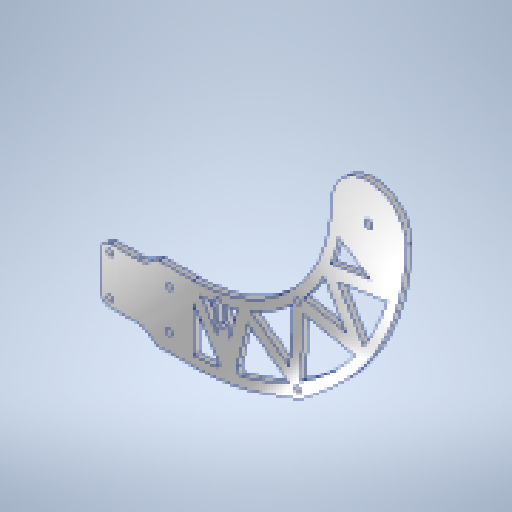
# Autodesk Inventor part: link1plate5
Saved by Autodesk Inventor 2024 (Build 280153000, 153)
## iProperties
Created: 2025-02-12
Part Number: link1plate5
Material: アルミニウム 6061
Document SubType Name: Modeling
Designer: tanoue_kota
Density: 2.7 g/cm^3
Appearance: アルミニウム - フラット
Mass: 39.1367 g
Surface Area: 135.061 cm^2
Volume: 14.4951 cm^3
Author: tanoue_kota
Autodesk Inventor part; units mm, degrees
ref_plane "YZ Plane" through (0, 0, 0) normal (1, 0, 0) x (0, 1, 0)
ref_plane "XZ Plane" through (0, 0, 0) normal (0, 1, 0) x (-1, 0, 0)
ref_plane "XY Plane" through (0, 0, 0) normal (0, 0, 1) x (1, 0, 0)
sketch "スケッチ1" plane through (0, 0, 0) normal (0, 0, 1) x (1, 0, 0)
  line L0 (0, 0) -> (-413, 0)
  line L1 (-413, 0) -> (-413, 19)
  line L2 (-413, 19) -> (0, 19)
  line L3 (0, 19) -> (0, 0)
  line L4 (-12.5, 0) -> (-47.5, 0)
  line L5 (-47.5, 0) -> (-47.5, 19)
  line L6 (-47.5, 19) -> (-12.5, 19)
  line L7 (-12.5, 19) -> (-12.5, 0)
  circle A0 centre (-413, 0) radius 510
  line L8 (-413, 0) -> (89.252, 88.5606)
  line L9 (89.252, 88.5606) -> (-410.748, 88.5606)
  line L10 (0, 0) -> (-20, 0)
  line L11 (-20, 0) -> (-20, 53.1786)
  line L12 (-20, 53.1786) -> (0, 53.1786)
  line L13 (0, 53.1786) -> (0, 0)
  line L14 (0, 53.1786) -> (-20, 53.1786)
  line L15 (-20, 53.1786) -> (-20, 88.5606)
  line L16 (-20, 88.5606) -> (0, 88.5606)
  line L17 (0, 88.5606) -> (0, 53.1786)
  circle A1 centre (89.252, 88.5606) radius 19
  line L18 (-413, -19) -> (0, -19)
  line L19 (0, -19) -> (0, 0)
  line L20 (-47.5, 0) -> (-47.5, -19)
  line L21 (-20, 0) -> (-20, -53.1786)
  line L22 (0, -53.1786) -> (0, 0)
  line L23 (0, -53.1786) -> (-20, -53.1786)
  line L24 (-413, 0) -> (-413, -19)
  arc A2 (0, 19) -> (70.2525, 88.7083) centre (0, 89.2547) ccw
  arc A3 (0, -19) -> (108.2514, 88.4128) centre (0, 89.2547) ccw
  line L25 (-47.5, 14) -> (-20, 14)
  line L26 (-47.5, -14) -> (-20, -14)
  line L27 (0, 88.5606) -> (6, 88.5606)
  line L28 (6, 88.5606) -> (6, 61.5606)
  line L29 (6, 61.5606) -> (0, 61.5606)
  line L30 (0, 61.5606) -> (0, 88.5606)
  line L31 (6, 88.5606) -> (57, 88.5606)
  line L32 (57, 88.5606) -> (57, 63.0606)
  line L33 (57, 63.0606) -> (6, 63.0606)
  line L34 (6, 63.0606) -> (6, 88.5606)
  line L35 (89.252, 88.5606) -> (0, 89.2547)
  point P0 (-20, 19)
  point P1 (-20, -14)
  point P2 (-20, -19)
  dimension "d4" = 1020
  dimension "d0" = 413
  dimension "d1" = 19
  dimension "d2" = 12.5
  dimension "d3" = 35
  dimension "d5" = 10
  dimension "d6" = 500
  dimension "d7" = 20
  dimension "d9" = 38
  dimension "d11" = 14
  dimension "d30" = 6
  dimension "d31" = 27
  dimension "d32" = 25.5
  dimension "d33" = 51
  dimension "d34" = 32.252
  dimension "d180" = 35.382
  dimension "d181" = 53.1786
  dimension "d187" = 89.554
  dimension "d188" = 89.2546
  dimension "d189" = 89.2519
  constraints: 72 end point, 12 parallel, 8 symmetric about line, 7 horizontal, 7 perpendicular, 7 point on line, 6 point on circle, 4 tangent, 3 centre point, 2 coincident, 3 other
  measures "d0" distance of L1.end L2.end
  measures "d1" distance of L2.end L0.start
  measures "d2" distance between parallel lines of L3 L7
  measures "d3" distance between parallel lines of L7 L5
  measures "d5" angle of L0 L8
  measures "d6" distance of L8.end L9.end
  measures "d7" distance between parallel lines of L13 L11
  measures "d9" diameter of A1
  measures "d11" distance between parallel lines of L4 L25
  measures "d30" distance between parallel lines of L17 L28
  measures "d31" distance of L27.end L28.end
  measures "d32" distance of L31.end L32.end
  measures "d33" distance of L32.end L33.end
  measures "d34" distance from line of L8.end L32
  measures "d180" distance between parallel lines of L9 L12
  measures "d181" distance between parallel lines of L0 L12
  measures "d187" angle of L30 L35
  measures "d188" distance of L0.start L35.end
  measures "d189" horizontal distance of L35.start L35.end
extrude "押し出し1" add sketch "スケッチ1" along normal blind 3 contours L19 L18 L21 L0 | L0 L7 L2 L3 | L3 A2 L8 A1 A0 A3 L19 | L0 L11 L2 L7 | L21 L26 L20 L0 | L0 L5 L25 L11 | A2 A1 L8 | A0 A1 A3 | A1 L9 L8 | L8 A0 A1 | A1 L35 L9 | A0 A1 | L35 A1 A0
sketch "スケッチ2" plane through (0, 0, 3) normal (0, 0, 1) x (1, 0, 0)
  arc A0 (108.2514, 88.4128) -> (70.2525, 88.7083) centre (89.252, 88.5606) ccw projected
  circle A1 centre (89.252, 88.5606) radius 2.1
  point P0 (0, 0)
  dimension "d16" = 4.2
  constraints: 1 centre point, 1 coincident
  measures "d16" diameter of A1
extrude "押し出し2" cut sketch "スケッチ2" against normal blind 3
sketch "スケッチ3" plane through (0, 0, 3) normal (0, 0, 1) x (1, 0, 0)
  line L0 (-20, 14) -> (-47.5, 14) projected
  line L1 (-42.5, 14) -> (-42.5, -14)
  line L2 (-47.5, -14) -> (-20, -14) projected
  line L3 (0, 19) -> (-20, 19) projected
  line L4 (-12.5, 19) -> (-12.5, -19)
  line L5 (-20, -19) -> (0, -19) projected
  line L6 (-47.5, 14) -> (-47.5, -14) projected
  line L7 (-47.5, 0) -> (0, 0)
  point P0 (-42.5, 10)
  point P1 (-12.5, 10)
  point P2 (-42.5, -10)
  point P3 (-12.5, -10)
  dimension "d19" = 5
  dimension "d20" = 30
  dimension "d21" = 10
  dimension "d22" = 10
  constraints: 6 end point, 6 point on line, 2 symmetric about line, 1 horizontal, 1 midpoint, 1 parallel, 1 vertical
  measures "d19" distance between parallel lines of L6 L1
  measures "d20" distance between parallel lines of L1 L4
  measures "d21" distance from line of L7 point (-42.5, 10)
  measures "d22" distance from line of L7 point (-12.5, 10)
hole "穴1" at (-42.5, 10, 3) at (-12.5, 10, 3) at (-42.5, -10, 3) at (-12.5, -10, 3) direction (0, 0, -1) diameter 3.1 end through all
sketch "スケッチ4" plane through (0, 0, 3) normal (0, 0, 1) x (1, 0, 0)
  line L0 (0, 19) -> (-20, 19) projected
  line L1 (0, 19) -> (0, -19)
  arc A0 (108.2514, 88.4128) -> (70.2525, 88.7083) centre (89.252, 88.5606) ccw projected
  arc A1 (0, -19) -> (108.2514, 88.4128) centre (0, 89.2547) ccw projected
  line L2 (70.2525, 88.7083) -> (108.2514, 88.4128)
  arc A2 (0, 19) -> (70.2525, 88.7083) centre (0, 89.2547) ccw projected
  line L3 (69.4594, 78.7142) -> (107.7108, 78.4167)
  arc A3 (0, 19) -> (70.2525, 88.7083) centre (0, 89.2547) ccw
  arc A4 (0, 14) -> (74.5073, 78.6749) centre (0, 89.2547) ccw
  arc A5 (0, -14) -> (102.6884, 78.4558) centre (0, 89.2547) ccw
  line L4 (0, 89.2547) -> (17.93, -12.4313)
  line L5 (0, 89.2547) -> (0, -19)
  line L6 (0, 89.2547) -> (35.3152, -7.773)
  line L7 (0, 89.2547) -> (51.6273, -0.1665)
  line L8 (0, 89.2547) -> (108.2514, 88.4128)
  line L9 (0, 89.2547) -> (73.0121, 16.2426)
  line L10 (0, 89.2547) -> (84.5813, 30.0302)
  line L11 (84.5813, 30.0302) -> (53.2131, 36.0416)
  line L12 (53.2131, 36.0416) -> (51.6273, -0.1665)
  line L13 (51.6273, -0.1665) -> (25.7386, 18.5384)
  line L14 (25.7386, 18.5384) -> (17.93, -12.4313)
  line L15 (0, 14) -> (17.93, -12.4313)
  circle A6 centre (89.252, 88.5606) radius 2.1 projected
  line L16 (0, 8.656) -> (14.6595, -12.9541)
  line L17 (3.5677, 14.0846) -> (21.1361, -11.8136)
  line L18 (22.3085, 17.3826) -> (14.6595, -12.9541)
  line L19 (29.1231, 19.8637) -> (21.1361, -11.8136)
  line L20 (22.3085, 17.3826) -> (48.786, -1.7478)
  line L21 (29.1231, 19.8637) -> (54.4805, 1.5426)
  line L22 (48.786, -1.7478) -> (50.3209, 33.2987)
  line L23 (54.4805, 1.5426) -> (56.1264, 39.1239)
  line L24 (50.3209, 33.2987) -> (82.479, 27.136)
  line L25 (56.1264, 39.1239) -> (86.7501, 33.2552)
  line L26 (14.6595, -12.9541) -> (9.7939, 14.64)
  line L27 (21.1361, -11.8136) -> (16.2706, 15.78)
  line L28 (0, 89.2547) -> (93.5805, 45.6174)
  line L29 (0, 89.2547) -> (99.7363, 62.5304)
  line L30 (84.5813, 30.0302) -> (68.2039, 57.4507)
  line L31 (68.2039, 57.4507) -> (99.7363, 62.5304)
  line L32 (74.5073, 78.6749) -> (99.7363, 62.5304)
  line L33 (82.479, 27.136) -> (66.4615, 53.954)
  line L34 (86.7501, 33.2552) -> (69.9219, 61.4305)
  line L35 (66.4615, 53.954) -> (98.7713, 59.1589)
  line L36 (69.9219, 61.4305) -> (100.6906, 66.3871)
  line L37 (98.7713, 59.1589) -> (73.9059, 75.0708)
  line L38 (100.6906, 66.3871) -> (81.5744, 78.62)
  point P0 (0, 0)
  point P1 (70.2525, 88.7083)
  point P2 (12.1996, 20.0673)
  point P3 (55.8251, 32.2439)
  point P4 (49.1004, 5.4298)
  point P5 (27.5438, 13.6)
  point P6 (18.5891, 2.6311)
  point P7 (12.113, 1.4877)
  point P8 (0, 8.656)
  point P9 (90.1335, 64.6864)
  point P10 (73.6917, 55.1187)
  point P11 (77.7997, 34.9704)
  point P12 (89.252, 88.5606)
  dimension "d136" = 5
  dimension "d137" = 5
  dimension "d138" = 10
  dimension "d139" = 75.2546
  dimension "d140" = 10
  dimension "d141" = 10
  dimension "d142" = 15
  dimension "d144" = 10
  dimension "d145" = 3
  dimension "d146" = 3
  dimension "d162" = 10
  dimension "d163" = 10
  dimension "d164" = 10
  dimension "d165" = 89.2519
  constraints: 76 end point, 19 parallel, 9 point on line, 4 point on circle, 3 coincident, 1 centre point, 1 collinear, 1 midpoint, 1 vertical, 36 other
  measures "d138" angle of L5 L4
  measures "d139" distance of A1.centre L15.start
  measures "d140" angle of L4 L6
  measures "d141" angle of L6 L7
  measures "d142" angle of L7 L9
  measures "d144" distance from line of L3 A6.centre
  measures "d145" distance between parallel lines of L15 L17
  measures "d146" distance between parallel lines of L15 L16
  measures "d162" angle of L9 L10
  measures "d163" angle of L10 L28
  measures "d164" angle of L28 L29
  measures "d165" horizontal distance of A3.centre point (89.252, 88.561)
extrude "押し出し3" cut sketch "スケッチ4" against normal blind 3 contours L16 A5 L1 | A4 L26 L17 | A4 L18 L27 | L7 L21 A4 | A4 L22 L21 L7 | L10 L25 A4 | A4 L33 L25 L10 | L29 L37 L36 A4 | A4 L37 L29 | L19 L6 A5 | L19 L20 A5 L6 | L24 A5 L9 | L9 A5 L23 L24 | L34 L35 A5 L28 | L28 A5 L34
sketch "スケッチ5" plane through (0, 0, 0) normal (0, 0, -1) x (-1, 0, 0)
  circle A0 centre (-89.252, 88.5606) radius 2.1 projected
  circle A1 centre (-89.252, 88.5606) radius 11
  circle A2 centre (-89.252, 88.5606) radius 7
  point P0 (0, 0)
  dimension "d59" = 22
  dimension "d60" = 14
  constraints: 2 centre point, 2 coincident
  measures "d59" diameter of A1
  measures "d60" diameter of A2
extrude "押し出し4" cut sketch "スケッチ5" against normal blind 0.5 contours A1
fillet "フィレット3" radius 10 2 edges at (-20, 14, 1.5) (-20, -14, 1.5)
fillet "フィレット4" radius 5 4 edges at (-47.5, 14, 1.5) (-47.5, -14, 1.5) (-20, -19, 1.5) (-20, 19, 1.5)
sketch "スケッチ11" plane through (0, 0, 3) normal (0, 0, 1) x (1, 0, 0)
  line L0 (-17.4799, -19) -> (0, -19) projected
  arc A0 (0, 19) -> (70.2525, 88.7083) centre (0, 89.2547) ccw projected
  line L1 (12.1765, 20.0633) -> (18.7751, -17.3594)
  arc A1 (0, -19) -> (108.2514, 88.4128) centre (0, 89.2547) ccw projected
  line L2 (9.7939, 14.64) -> (12.113, 1.4877) projected
  line L3 (12.113, 1.4877) -> (18.5891, 2.6311)
  circle A2 centre (0, 89.2547) radius 0.0235
  circle A3 centre (0, 89.2547) radius 74
  circle A4 centre (0, 89.2547) radius 84
  circle A5 centre (12.8268, 16.3748) radius 1.55
  circle A6 centre (14.5633, 6.5267) radius 1.55
  line L4 (11.2976, 16.1221) -> (13.0344, 6.2721)
  line L5 (14.3505, 16.6594) -> (16.0873, 6.8095)
  point P0 (0, 0)
  point P1 (15.351, 2.0594)
  point P2 (14.3559, 16.6284)
  point P3 (11.3034, 16.0892)
  dimension "d149" = 3.1
  dimension "d150" = 3.1
  dimension "d160" = 148
  dimension "d161" = 168
  constraints: 12 point on circle, 8 end point, 5 centre point, 3 coincident, 3 point on line, 1 midpoint, 1 parallel, 1 tangent
  measures "d149" diameter of A5
  measures "d150" diameter of A6
  measures "d160" diameter of A3
  measures "d161" diameter of A4
extrude "押し出し6" cut sketch "スケッチ11" against normal blind 3 contours A5 A3 L1 | L1 A3 A5 | A3 L5 A6 L1 | L1 A5 A3 | A5 L1 A6 L4 | A6 L1 A4 | A4 L1 A6 | A6 L1 A4 | A4 L1 A6
sketch "スケッチ13" plane through (0, 0, 3) normal (0, 0, 1) x (1, 0, 0)
  arc A0 (0, 19) -> (70.2525, 88.7083) centre (0, 89.2547) ccw projected
  arc A1 (0, -19) -> (108.2514, 88.4128) centre (0, 89.2547) ccw projected
  circle A2 centre (0, 89.2547) radius 104
  circle A3 centre (0, 89.2547) radius 75
  line L0 (86.7501, 33.2552) -> (73.6917, 55.1187) projected
  line L1 (0, 89.2547) -> (0, -14.7453)
  line L2 (0, 89.2547) -> (73.5391, 15.7155)
  point P0 (0, 0)
  point P1 (49.1004, 5.4298)
  point P2 (55.8251, 32.2439)
  point P3 (53.033, 36.2216)
  dimension "d152" = 150
  dimension "d151" = 208
  dimension "d177" = 45
  constraints: 4 end point, 2 coincident, 2 point on circle, 1 centre point, 1 point on line, 1 vertical, 3 other
  measures "d151" diameter of A2
  measures "d177" angle of L1 L2
hole "穴7" at (53.033, 36.2216, 3) direction (0, 0, -1) diameter 3.1 end through all
sketch "スケッチ14" plane through (0, 0, 3) normal (0, 0, 1) x (1, 0, 0)
  arc A0 (0, 19) -> (70.2525, 88.7083) centre (0, 89.2547) ccw projected
  arc A1 (0, -19) -> (108.2514, 88.4128) centre (0, 89.2547) ccw projected
  line L0 (0, 89.2547) -> (0, -19)
  circle A2 centre (0, 89.2547) radius 108.2547
  line L1 (55, -6.0081) -> (0, 89.2547)
  line L2 (55, -6.0081) -> (36.6341, -12.613)
  line L3 (55, -6.0081) -> (69.9029, 6.5948)
  point P0 (0, 0)
  point P1 (69.9029, 6.5948)
  point P2 (36.6341, -12.613)
  dimension "d182" = 110
  dimension "d183" = 30
  constraints: 8 end point, 3 point on circle, 2 tangent, 1 centre point, 1 coincident, 1 vertical
  measures "d182" distance of L1.start L1.end
  measures "d183" angle of L0 L1
extrude "押し出し7" add sketch "スケッチ14" against normal blind 3 contours L1 L2 A1 | A1 L3 L1
sketch "スケッチ15" plane through (0, 0, 3) normal (0, 0, 1) x (1, 0, 0)
  arc A0 (0, 19) -> (70.2525, 88.7083) centre (0, 89.2547) ccw projected
  line L0 (0, 89.2547) -> (0, -19)
  line L1 (-17.4799, -19) -> (0, -19) projected
  line L2 (53, -2.544) -> (0, 89.2547)
  point P0 (0, 0)
  dimension "d184" = 30
  dimension "d185" = 106
  constraints: 5 end point, 1 vertical
  measures "d184" angle of L0 L2
  measures "d185" distance of L2.start L0.start
hole "穴8" at (53, -2.544, 3) direction (0, 0, -1) diameter 3.1 end through all
fillet "フィレット6" radius 2 2 edges at (21.1361, -11.8136, 1.5) (14.6595, -12.9541, 1.5)
